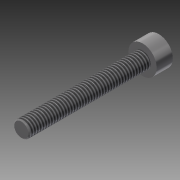
# Autodesk Inventor part: SHCS4x30
Saved by Autodesk Inventor 2015 SP1 (Build 190203100, 203)
## iProperties
Category: Hardware
Created: 2013-12-08
Part Number: SHCS4x30
Material: Stainless Steel
Document SubType Name: Modeling
Designer: Jack
Density: 8 g/cm^3
Appearance: Semi-Polished
Mass: 4.03159 g
Surface Area: 5.73258 cm^2
Volume: 0.503949 cm^3
Vendor: Misumi
Author: Jack
Title: SHCS 4x30
Autodesk Inventor part; units mm, degrees
ref_plane "YZ Plane" through (0, 0, 0) normal (1, 0, 0) x (0, 1, 0)
ref_plane "XZ Plane" through (0, 0, 0) normal (0, 1, 0) x (-1, 0, 0)
ref_plane "XY Plane" through (0, 0, 0) normal (0, 0, 1) x (1, 0, 0)
sketch "Sketch1" plane through (0, 0, 0) normal (0, 1, 0) x (-1, 0, 0)
  circle A0 centre (0, 0) radius 2
  dimension "d0" = 4
  constraints: 1 centre point, 1 coincident
  measures "d0" diameter of A0
extrude "Extrusion1" add sketch "Sketch1" along normal blind 30
sketch "Sketch2" plane through (0, 30, 0) normal (0, 1, 0) x (1, 0, 0)
  circle A0 centre (0, 0) radius 2 projected
  circle A1 centre (0, 0) radius 3.5
  dimension "d3" = 7
  constraints: 1 centre point, 1 coincident
  measures "d3" diameter of A1
extrude "Extrusion2" add sketch "Sketch2" along normal blind 4 contours A0 | A1
sketch "Sketch3" plane through (0, 34, 0) normal (0, 1, 0) x (1, 0, 0)
  circle A0 centre (0, 0) radius 3.5 projected
  line L0 (0, 1.8475) -> (1.6, 0.9238)
  line L1 (1.6, 0.9238) -> (1.6, -0.9238)
  line L2 (1.6, -0.9238) -> (0, -1.8475)
  line L3 (0, -1.8475) -> (-1.6, -0.9238)
  line L4 (-1.6, -0.9238) -> (-1.6, 0.9238)
  line L5 (-1.6, 0.9238) -> (0, 1.8475)
  dimension "d6" = 1.6
  constraints: 12 end point, 1 coincident, 1 vertical, 13 other
  measures "d6" distance from line of L1 point (0, 0)
extrude "Extrusion3" cut sketch "Sketch3" against normal blind 3 contours L0 L1 L2 L3 L4 L5
thread "Thread1" size "M4x0.7" class "6g" standard "ANSI Metric M Profile" full length
chamfer "Chamfer1" distance 0.25 angle 45 1 edges at (2, 0, 0)
body "Solid1"
